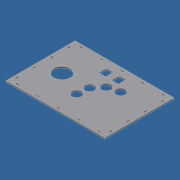
# Autodesk Inventor part: P1704_021_dessus_manette
Saved by Autodesk Inventor 2019 (Build 230136000, 136)
## iProperties
Created: 2019-06-21
Part Number: P1704_021_dessus_manette
Project: Nom Projet
Material: .
Description: Nom pièce
Document SubType Name: Modeling
Designer: Adel.KAHRIMANOVIC
Authority: brut Ø
Density: 0.001 g/cm^3
Appearance: Par défaut
Material number: ---
Author: Adel.KAHRIMANOVIC
Autodesk Inventor part; units mm, degrees
ref_plane "Plan YZ" through (0, 0, 0) normal (1, 0, 0) x (0, 1, 0)
ref_plane "Plan XZ" through (0, 0, 0) normal (0, 1, 0) x (-1, 0, 0)
ref_plane "Plan XY" through (0, 0, 0) normal (0, 0, 1) x (1, 0, 0)
sketch "Esquisse1" plane through (0, 0, 0) normal (0, 0, 1) x (1, 0, 0)
  line L0 (0, 0) -> (300, 0)
  line L1 (300, 0) -> (300, 210)
  line L2 (300, 210) -> (0, 210)
  line L3 (0, 210) -> (0, 0)
  dimension "d0" = 300
  dimension "d1" = 210
  constraints: 8 end point, 2 parallel, 1 horizontal, 1 perpendicular
  measures "d0" distance of L0.start L0.end
  measures "d1" distance of L2.end L0.start
extrude "Extrusion1" add sketch "Esquisse1" along normal blind 4
sketch "Esquisse6" plane through (0, 0, 4) normal (0, 0, 1) x (1, 0, 0)
  line L0 (6, 20) -> (10, 20)
  line L1 (10, 20) -> (10, 32)
  line L2 (10, 32) -> (6, 32)
  line L3 (6, 32) -> (6, 20)
  line L4 (0, 210) -> (0, 0) projected
  line L5 (6, 72.6667) -> (10, 72.6667)
  line L6 (10, 72.6667) -> (10, 84.6667)
  line L7 (10, 84.6667) -> (6, 84.6667)
  line L8 (6, 84.6667) -> (6, 72.6667)
  line L9 (6, 125.3333) -> (10, 125.3333)
  line L10 (10, 125.3333) -> (10, 137.3333)
  line L11 (10, 137.3333) -> (6, 137.3333)
  line L12 (6, 137.3333) -> (6, 125.3333)
  line L13 (6, 178) -> (10, 178)
  line L14 (10, 178) -> (10, 190)
  line L15 (10, 190) -> (6, 190)
  line L16 (6, 190) -> (6, 178)
  line L17 (0, 0) -> (300, 0) projected
  line L18 (300, 210) -> (0, 210) projected
  line L19 (8, 32) -> (8, 72.6667) construction
  line L20 (8, 178) -> (8, 137.3333) construction
  line L21 (8, 84.6667) -> (8, 125.3333) construction
  line L22 (300, 0) -> (0, 210) construction
  line L23 (20, 6) -> (32, 6)
  line L24 (32, 6) -> (32, 10)
  line L25 (32, 10) -> (20, 10)
  line L26 (20, 10) -> (20, 6)
  line L27 (82, 6) -> (94, 6)
  line L28 (94, 6) -> (94, 10)
  line L29 (94, 10) -> (82, 10)
  line L30 (82, 10) -> (82, 6)
  line L31 (206, 6) -> (218, 6)
  line L32 (218, 6) -> (218, 10)
  line L33 (218, 10) -> (206, 10)
  line L34 (206, 10) -> (206, 6)
  line L35 (268, 6) -> (280, 6)
  line L36 (280, 6) -> (280, 10)
  line L37 (280, 10) -> (268, 10)
  line L38 (268, 10) -> (268, 6)
  line L39 (300, 0) -> (300, 210) projected
  line L40 (268, 8) -> (218, 8) construction
  line L41 (82, 8) -> (32, 8) construction
  line L42 (144, 6) -> (156, 6)
  line L43 (156, 6) -> (156, 10)
  line L44 (156, 10) -> (144, 10)
  line L45 (144, 10) -> (144, 6)
  line L46 (206, 8) -> (156, 8) construction
  line L47 (144, 8) -> (94, 8) construction
  line L48 (300, 210) -> (0, 0) construction
  line L49 (150, 105) -> (150, 157.6667) construction
  line L50 (150, 105) -> (99.3471, 105) construction
  line L51 (20, 204) -> (32, 204)
  line L52 (32, 204) -> (32, 200)
  line L53 (32, 200) -> (20, 200)
  line L54 (20, 200) -> (20, 204)
  line L55 (82, 204) -> (94, 204)
  line L56 (94, 204) -> (94, 200)
  line L57 (94, 200) -> (82, 200)
  line L58 (82, 200) -> (82, 204)
  line L59 (206, 204) -> (218, 204)
  line L60 (218, 204) -> (218, 200)
  line L61 (218, 200) -> (206, 200)
  line L62 (206, 200) -> (206, 204)
  line L63 (268, 204) -> (280, 204)
  line L64 (280, 204) -> (280, 200)
  line L65 (280, 200) -> (268, 200)
  line L66 (268, 200) -> (268, 204)
  line L67 (268, 202) -> (218, 202) construction
  line L68 (82, 202) -> (32, 202) construction
  line L69 (144, 204) -> (156, 204)
  line L70 (156, 204) -> (156, 200)
  line L71 (156, 200) -> (144, 200)
  line L72 (144, 200) -> (144, 204)
  line L73 (206, 202) -> (156, 202) construction
  line L74 (144, 202) -> (94, 202) construction
  line L75 (294, 20) -> (290, 20)
  line L76 (290, 20) -> (290, 32)
  line L77 (290, 32) -> (294, 32)
  line L78 (294, 32) -> (294, 20)
  line L79 (294, 72.6667) -> (290, 72.6667)
  line L80 (290, 72.6667) -> (290, 84.6667)
  line L81 (290, 84.6667) -> (294, 84.6667)
  line L82 (294, 84.6667) -> (294, 72.6667)
  line L83 (294, 125.3333) -> (290, 125.3333)
  line L84 (290, 125.3333) -> (290, 137.3333)
  line L85 (290, 137.3333) -> (294, 137.3333)
  line L86 (294, 137.3333) -> (294, 125.3333)
  line L87 (294, 178) -> (290, 178)
  line L88 (290, 178) -> (290, 190)
  line L89 (290, 190) -> (294, 190)
  line L90 (294, 190) -> (294, 178)
  line L91 (292, 32) -> (292, 72.6667) construction
  line L92 (292, 178) -> (292, 137.3333) construction
  line L93 (292, 84.6667) -> (292, 125.3333) construction
  dimension "d4" = 4
  dimension "d6" = 20
  dimension "d7" = 20
  dimension "d8" = 6
  dimension "d9" = 12
  dimension "d10" = 20
  dimension "d11" = 20
  dimension "d12" = 12
  dimension "d13" = 6
  dimension "d14" = 4
  constraints: 180 end point, 50 symmetric about line, 20 point on line, 18 parallel, 15 midpoint, 13 equal length, 10 horizontal, 9 perpendicular, 3 collinear, 1 vertical
  measures "d4" distance between parallel lines of L3 L1
  measures "d6" distance between parallel lines of L0 L17
  measures "d7" distance between parallel lines of L18 L15
  measures "d8" distance between parallel lines of L4 L3
  measures "d9" distance between parallel lines of L0 L2
  measures "d10" distance between parallel lines of L4 L26
  measures "d11" distance between parallel lines of L39 L36
  measures "d12" distance between parallel lines of L36 L38
  measures "d13" distance between parallel lines of L17 L23
  measures "d14" distance between parallel lines of L27 L29
extrude "Extrusion2" cut sketch "Esquisse6" against normal blind 4 contours L3 L2 L1 L0 | L8 L7 L6 L5 | L12 L11 L10 L9 | L16 L15 L14 L13 | L26 L25 L24 L23 | L30 L29 L28 L27 | L34 L33 L32 L31 | L38 L37 L36 L35 | L45 L44 L43 L42 | L51 L52 L53 L54 | L55 L56 L57 L58 | L59 L60 L61 L62 | L63 L64 L65 L66 | L69 L70 L71 L72 | L75 L76 L77 L78 | L79 L80 L81 L82 | L83 L84 L85 L86 | L87 L88 L89 L90
sketch "Esquisse8" plane through (0, 0, 4) normal (0, 0, 1) x (1, 0, 0)
  line L0 (0, 210) -> (0, 0) projected
  line L1 (300, 210) -> (0, 210) projected
  point P0 (10, 200)
  dimension "d39" = 10
  dimension "d40" = 10
  measures "d39" distance from line of L0 point (10, 200)
  measures "d40" distance from line of point (10, 200) L1
hole "Perçage2" at (10, 200, 4) direction (0, 0, -1) diameter 3.4 end through all counterbore diameter 6.5 counterbore depth 2
pattern_linear "Réseau rectangulaire2" count 2 spacing 190 along (0, -1, 0) count 2 spacing 280 along (1, 0, 0) of "Perçage2"
sketch "Esquisse10" plane through (0, 0, 4) normal (0, 0, 1) x (1, 0, 0)
  circle A0 centre (65, 105) radius 24.75
  line L0 (300, 210) -> (0, 210) projected
  line L1 (-375.2445, 105) -> (140.113, 105) construction
  line L2 (-117.5657, 105) -> (-117.5657, 0) construction
  line L3 (-117.5657, 105) -> (-117.5657, 210) construction
  line L4 (0, 0) -> (300, 0) construction
  line L5 (0, 210) -> (0, 0) construction
  dimension "d64" = 49.5
  dimension "d66" = 65
  constraints: 6 end point, 3 point on line, 2 vertical, 1 centre point, 1 collinear, 1 horizontal, 1 midpoint
  measures "d64" diameter of A0
  measures "d66" distance from line of L5 A0.centre
extrude "Extrusion3" cut sketch "Esquisse10" against normal blind 4
sketch "Esquisse9" plane through (0, 0, 4) normal (0, 0, 1) x (1, 0, 0)
  circle A0 centre (65, 105) radius 24.75 projected
  point P0 (0, 0)
  point P1 (42.5, 127.5)
  dimension "d62" = 22.5
  dimension "d63" = 22.5
  measures "d62" horizontal distance of point (42.5, 127.5) A0.centre
  measures "d63" horizontal distance of A0.centre point (42.5, 127.5)
hole "Perçage3" at (42.5, 127.5, 4) direction (0, 0, -1) diameter 2.9 end through all counterbore diameter 5.5 counterbore depth 2
pattern_linear "Réseau rectangulaire3" count 2 spacing 45 along (1, 0, 0) count 2 spacing 45 along (0, -1, 0) of "Perçage3"
sketch "Esquisse11" plane through (0, 0, 4) normal (0, 0, 1) x (1, 0, 0)
  line L0 (120.3, 185) -> (141, 185)
  line L1 (141, 185) -> (141, 161.6)
  line L2 (141, 161.6) -> (120.3, 161.6)
  line L3 (120.3, 161.6) -> (120.3, 185)
  line L4 (159, 185) -> (179.7, 185)
  line L5 (179.7, 185) -> (179.7, 161.6)
  line L6 (179.7, 161.6) -> (159, 161.6)
  line L7 (159, 161.6) -> (159, 185)
  line L8 (300, 210) -> (0, 210) projected
  line L9 (0, 171.6331) -> (120.3, 171.6331) construction
  line L10 (179.7, 173.3) -> (300, 173.3) construction
  line L11 (300, 0) -> (300, 210) projected
  line L12 (0, 210) -> (0, 0) projected
  dimension "d67" = 23.4
  dimension "d68" = 20.7
  dimension "d69" = 18
  dimension "d70" = 25
  constraints: 20 end point, 4 parallel, 3 horizontal, 3 perpendicular, 3 point on line, 2 collinear, 2 equal length, 1 midpoint
  measures "d67" distance between parallel lines of L2 L0
  measures "d68" distance of L0.start L0.end
  measures "d69" distance between parallel lines of L7 L1
  measures "d70" distance between parallel lines of L8 L0
extrude "Extrusion4" cut sketch "Esquisse11" against normal blind 4
sketch "Esquisse12" plane through (0, 0, 4) normal (0, 0, 1) x (1, 0, 0)
  circle A0 centre (203.8181, 144.2332) radius 14
  circle A1 centre (146.095, 108.1212) radius 14
  circle A2 centre (142.2966, 72.6698) radius 14
  circle A3 centre (169.338, 135.1581) radius 14
  arc A4 (189.5373, 25.4286) -> (174.5392, 30.5211) centre (201.1601, 84.2921) ccw construction
  line L0 (300, 0) -> (300, 210) projected
  line L1 (0, 0) -> (300, 0) projected
  line L2 (203.8181, 144.2332) -> (169.338, 135.1581) construction
  line L3 (146.095, 108.1212) -> (169.338, 135.1581) construction
  line L4 (142.2966, 72.6698) -> (146.095, 108.1212) construction
  dimension "d77" = 28
  dimension "d80" = 60
  constraints: 6 end point, 6 point on circle, 5 centre point, 3 equal radius, 2 equal length
  measures "d77" diameter of A2
  measures "d80" radius of A4
extrude "Extrusion5" cut sketch "Esquisse12" against normal blind 4
